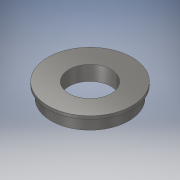
# Autodesk Inventor part: F6805ZZ
Saved by Autodesk Inventor 2019.4 (Build 234330000, 330)
## iProperties
Created: 2019-12-07
Part Number: F6805ZZ
Material: Stainless Steel
Document SubType Name: Modeling
Designer: admin
Density: 8 g/cm^3
Appearance: Semi-Polished
Author: admin
Autodesk Inventor part; units mm, degrees
ref_plane "YZ Plane" through (0, 0, 0) normal (1, 0, 0) x (0, 1, 0)
ref_plane "XZ Plane" through (0, 0, 0) normal (0, 1, 0) x (-1, 0, 0)
ref_plane "XY Plane" through (0, 0, 0) normal (0, 0, 1) x (1, 0, 0)
sketch "Sketch1" plane through (0, 0, 0) normal (0, 0, 1) x (1, 0, 0)
  line L0 (-20, 7) -> (-20, 5.5)
  line L1 (-20, 5.5) -> (-18.5, 5.5)
  line L2 (-18.5, 5.5) -> (-18.5, 0)
  line L3 (-18.5, 0) -> (-10, 0)
  line L4 (-10, 0) -> (-10, 7)
  line L5 (-10, 7) -> (-20, 7)
  line L6 (0, 0) -> (0, 8.0623) construction
  dimension "d0" = 7
  dimension "d1" = 18.5
  dimension "d2" = 10
  dimension "d3" = 20
  dimension "d4" = 1.5
  constraints: 14 end point, 5 perpendicular, 2 vertical, 1 point on line
  measures "d0" distance of L3.end L4.end
  measures "d1" distance of L6.start L2.end
  measures "d2" distance from line of L6.start L4
  measures "d3" distance from line of L6.start L0
  measures "d4" distance of L0.start L0.end
revolve "Revolution1" add sketch "Sketch1" angle 360 about axis through (0, 0, 0) along (0, 1, 0)
body "Solid1"
